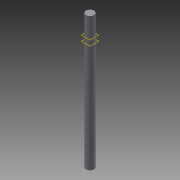
# Autodesk Inventor part: input_spindle
Saved by Autodesk Inventor 2014 (Build 180170000, 170)
## iProperties
Created: 2015-06-18
Part Number: input_spindle
Material: Generic
Document SubType Name: Modeling
Designer: vorac
Density: 1 g/cm^3
Appearance: Default
Author: vorac
Autodesk Inventor part; units mm, degrees
ref_plane "YZ Plane" through (0, 0, 0) normal (1, 0, 0) x (0, 1, 0)
ref_plane "XZ Plane" through (0, 0, 0) normal (0, 1, 0) x (-1, 0, 0)
ref_plane "XY Plane" through (0, 0, 0) normal (0, 0, 1) x (1, 0, 0)
sketch "Sketch1" plane through (0, 0, 0) normal (0, 0, 1) x (1, 0, 0)
  circle A0 centre (0, 0) radius 14.9305
  line L0 (4.7107, 14.1679) -> (-4.7107, 14.1679)
  line L1 (-4.7107, 14.1679) -> (-4.7107, 10.3691)
  line L2 (-4.7107, 10.3691) -> (4.7107, 10.3691)
  line L3 (4.7107, 10.3691) -> (4.7107, 14.1679)
  line L4 (0, 0) -> (0, 27.3143) construction
  point P0 (0, 10.3691)
  dimension "d0" = 29.861
  dimension "d3" = 3.7988
  dimension "d4" = 9.4214
  constraints: 10 end point, 3 perpendicular, 2 point on circle, 1 centre point, 1 coincident, 1 midpoint, 1 point on line, 1 vertical
  measures "d0" diameter of A0
  measures "d3" distance of L2.end L0.start
  measures "d4" distance of L0.start L0.end
extrude "Extrusion1" add sketch "Sketch1" along normal blind 500
sketch "Sketch2" plane through (0, 0, 500) normal (0, 0, 1) x (1, 0, 0)
  circle A0 centre (0, 0) radius 14.9305 projected
  line L0 (-3.4258, 14.5322) -> (-3.4258, 10.4702)
  line L1 (-3.4258, 10.4702) -> (3.4258, 10.4702)
  line L2 (3.4258, 10.4702) -> (3.4258, 14.5322)
  line L3 (0, 0) -> (0, 23.7293) construction
  point P0 (0, 10.4702)
  dimension "d5" = 4.0619
  dimension "d6" = 6.8516
  constraints: 8 end point, 2 perpendicular, 2 point on circle, 1 horizontal, 1 midpoint, 1 parallel, 1 point on line
  measures "d5" distance of L1.end L2.end
  measures "d6" distance of L0.end L1.end
ref_plane "Work Plane1" through (0, 0, 428) normal (0, 0, 1) x (1, 0, 0)
ref_plane "Work Plane2" through (0, 0, 408.25) normal (0, 0, 1) x (1, 0, 0)
extrude "Extrusion2" cut sketch "Sketch2" against normal up to surface (19.75 mm away) from surface at -72 contours L2 L1 L0 A0 picked at (0.3837, 11.9422)
body "Solid1"
